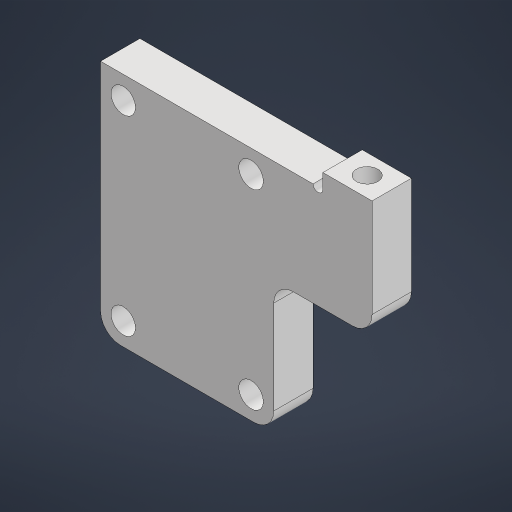
# Autodesk Inventor part: SolenoidMount
Saved by Autodesk Inventor 2024.2 (Build 282272000, 272)
## iProperties
Created: 2023-12-22
Part Number: SolenoidMount
Material: 一般
Document SubType Name: Modeling
Designer: Hanaoka
Density: 1 g/cm^3
Appearance: 既定
Author: Hanaoka
Autodesk Inventor part; units mm, degrees
ref_plane "YZ Plane" through (0, 0, 0) normal (1, 0, 0) x (0, 1, 0)
ref_plane "XZ Plane" through (0, 0, 0) normal (0, 1, 0) x (-1, 0, 0)
ref_plane "XY Plane" through (0, 0, 0) normal (0, 0, 1) x (1, 0, 0)
ref_plane "作業平面1" through (0, 0, 0) normal (0, 0, 1) x (1, 0, 0)
sketch "スケッチ1" plane through (0, 0, 0) normal (0, 0, 1) x (1, 0, 0)
  line L0 (0, -24) -> (-27.3, -24) projected
  line L1 (-3.7, -24) -> (-3.7, -10.5)
  line L2 (-3.7, -10.5) -> (6.3, -10.5)
  line L3 (6.3, -10.5) -> (6.3, 1.5)
  line L4 (6.3, 1.5) -> (1.3, 1.5)
  line L5 (-27.3, 0) -> (0, 0) projected
  line L6 (1.3, 1.5) -> (1.3, 0)
  circle A0 centre (-6, -21.7) radius 1.25 projected
  circle A1 centre (-19, -21.7) radius 1.25 projected
  circle A2 centre (-6, -21.7) radius 2.3 construction
  circle A3 centre (-19, -21.7) radius 2.3 construction
  line L7 (1.3, 0) -> (0, 0)
  line L8 (-21.3, -24) -> (-21.3, 0)
  circle A4 centre (-6, -2.3) radius 1.25 projected
  circle A5 centre (-19, -2.3) radius 1.25 projected
  line L9 (1.3, 0) -> (0.8, 0)
  arc A6 (0.3, 0) -> (1.3, 0) centre (0.8, 0) ccw
  dimension "d0" = 1.5
  dimension "d1" = 12
  dimension "d2" = 10
  dimension "d3" = 5
  dimension "d9" = 0.5
  constraints: 16 end point, 6 point on line, 4 tangent, 3 centre point, 3 coincident, 3 vertical, 2 horizontal, 2 point on circle, 1 collinear, 1 parallel
  measures "d0" distance of L4.end L6.end
  measures "d1" distance of L2.end L3.end
  measures "d2" distance of L1.end L2.end
  measures "d3" distance of L3.end L4.end
  measures "d9" distance of L6.end L9.end
extrude "押し出し1" add sketch "スケッチ1" along normal blind 4 contours L0 L8 L5 L7 A6 L6 L4 L3 L2 L1
sketch "スケッチ2" plane through (1.3, 1.5, 0) normal (0, 1, 0) x (1, 0, 0)
  line L0 (5, 0) -> (5, -4) projected
  line L1 (0, 0) -> (-22.6, 0) projected
  line L2 (5, -4) -> (0, 0) construction
  circle A0 centre (2.5, -2) radius 1.1
  point P0 (-1.3, 0)
  dimension "d6" = 2.2
  constraints: 2 end point, 1 centre point, 1 coincident, 1 midpoint
  measures "d6" diameter of A0
extrude "押し出し2" cut sketch "スケッチ2" against normal blind 5
fillet "フィレット1" radius 2 4 edges at (6.3, -10.5, 2) (-3.7, -10.5, 2) (-3.7, -24, 2) (-21.3, -24, 2)
